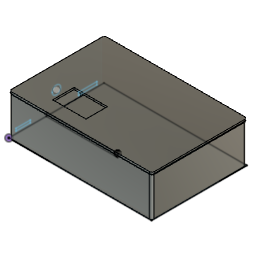
Ground Unit Enclosure v1.2 2 (Autodesk Fusion 360 design; units mm, degrees)
Autodesk Fusion 360 part; units mm, degrees
sketch "Sketch2" plane through (0, 0, 0) normal (0, 0, 1) x (1, 0, 0) in component "Case"
  line L0 (0, 0) -> (120, 0)
  line L1 (120, 0) -> (120, 80)
  line L2 (120, 80) -> (0, 80)
  line L3 (0, 80) -> (0, 0)
  dimension "d14" = 120
  dimension "d15" = 80
  constraint horizontal L0
  constraint vertical L1
  constraint horizontal L2
  constraint vertical L3
  constraint coincident L0.start L3.end
  measures "d14" distance of L0.start L0.end
  measures "d15" distance of L0.start L2.end
extrude "Extrude3" add sketch "Sketch2" along normal blind 33 makes body 1 in component "Case"
fillet "Fillet2" radius 2 1 edges at (120, 0, 16.5) on bodies 1 in component "Case"
fillet "Fillet3" radius 2 1 edges at (0, 0, 16.5) on bodies 1 in component "Case"
fillet "Fillet4" radius 2 2 edges at (120, 80, 16.5) (0, 80, 16.5) on bodies 1 in component "Case"
shell "Shell2" thickness 1.5 removed faces 1 at (40.6667, 26.6667, 33) on bodies 1 in component "Case"
sketch "Sketch Nub protrusion" plane through (0, 1.5, 0) normal (0, 1, 0) x (-1, 0, 0) in component "Case"
  line L0 (-2, 1.5) -> (-2, 33)
  line L1 (-2, 33) -> (-118, 33)
  line L2 (-118, 33) -> (-118, 1.5)
  line L3 (-118, 1.5) -> (-2, 1.5)
  line L4 (-90, 33) -> (-30, 33)
  line L5 (-30, 33) -> (-30, 30)
  line L6 (-30, 30) -> (-90, 30)
  line L7 (-90, 30) -> (-90, 33)
  line L8 (-60, 33) -> (-60, 30) construction
  dimension "d22" = 60
  dimension "d23" = 3
  constraint horizontal L4
  constraint vertical L5
  constraint horizontal L6
  constraint vertical L7
  constraint coincident L1 L4.start
  constraint midpoint L1 L8.start
  constraint midpoint L6 L8.end
  constraint vertical L8
  measures "d22" distance of L4.start L4.end
  measures "d23" distance of L4.start L6.end
extrude "Extrude4" add sketch "Sketch Nub protrusion" along normal blind 6 draft -45 contours L1 L4 L5 L6 L7 bodies 1 in component "Case"
ref_plane "WorkPlane1" through (60, 40, 16.5) normal (0, -1, 0) x (1, 0, 0) in component "Case"
mirror "Mirror1" about plane through (60, 40, 16.5) normal (0, -1, 0) of "Extrude4" in component "Case"
sketch "Sketch1" plane through (0, 0, 33) normal (0, 0, 1) x (-1, 0, 0) in component "Top Cover"
  arc A0 (-1.5, -2) -> (-2, -1.5) centre (-2, -2) ccw
  line L0 (-1.5, -2) -> (-1.5, -78)
  arc A1 (-2, -78.5) -> (-1.5, -78) centre (-2, -78) ccw
  line L1 (-2, -78.5) -> (-30, -78.5)
  line L2 (-30, -78.5) -> (-90, -78.5)
  line L3 (-90, -78.5) -> (-118, -78.5)
  arc A2 (-118.5, -78) -> (-118, -78.5) centre (-118, -78) ccw
  line L4 (-118.5, -78) -> (-118.5, -2)
  arc A3 (-118, -1.5) -> (-118.5, -2) centre (-118, -2) ccw
  line L5 (-118, -1.5) -> (-90, -1.5)
  line L6 (-90, -1.5) -> (-30, -1.5)
  line L7 (-30, -1.5) -> (-2, -1.5)
  arc A4 (-2, -80) -> (0, -78) centre (-2, -78) ccw
  line L8 (0, -78) -> (0, -2)
  arc A5 (0, -2) -> (-2, 0) centre (-2, -2) ccw
  line L9 (-2, 0) -> (-118, 0)
  arc A6 (-118, 0) -> (-120, -2) centre (-118, -2) ccw
  line L10 (-120, -2) -> (-120, -78)
  arc A7 (-120, -78) -> (-118, -80) centre (-118, -78) ccw
  line L11 (-118, -80) -> (-2, -80)
extrude "Extrude1" add sketch "Sketch1" along normal blind 2 separate body contours A0 L0 A1 L1 L2 L3 A2 L4 A3 L5 L6 L7 | A4 L8 A5 L9 A6 L10 A7 L11 makes body 2 in component "Top Cover"
sketch "Sketch2 (2)" plane through (0, 0, 33) normal (0, 0, -1) x (1, 0, 0) in component "Top Cover"
  line L0 (2, -80) -> (118, -80)
  arc A0 (118, -80) -> (120, -78) centre (118, -78) ccw
  line L1 (120, -78) -> (120, -2)
  arc A1 (120, -2) -> (118, 0) centre (118, -2) ccw
  line L2 (118, 0) -> (2, 0)
  arc A2 (2, 0) -> (0, -2) centre (2, -2) ccw
  line L3 (0, -2) -> (0, -78)
  arc A3 (0, -78) -> (2, -80) centre (2, -78) ccw
  arc A4 (1.7, -78) -> (2, -78.3) centre (2, -78) ccw
  line L4 (2, -78.3) -> (118, -78.3)
  arc A5 (118, -78.3) -> (118.3, -78) centre (118, -78) ccw
  line L5 (118.3, -78) -> (118.3, -2)
  arc A6 (118.3, -2) -> (118, -1.7) centre (118, -2) ccw
  line L6 (118, -1.7) -> (2, -1.7)
  arc A7 (2, -1.7) -> (1.7, -2) centre (2, -2) ccw
  line L7 (1.7, -2) -> (1.7, -78)
extrude "Extrude4'" add sketch "Sketch2 (2)" along normal blind 3 contours A4 L4 A5 L5 A6 L6 A7 L7 bodies 2 in component "Top Cover"
extrude "Extrude2" add sketch "Sketch2 (2)" along normal blind 3 contours A4 L4 A5 L5 A6 L6 A7 L7 bodies 2 in component "Top Cover"
extrude "Extrude3'" cut sketch "Sketch Nub protrusion" along normal blind 3 draft -45 from surface at 0.2 contours L1 L4 L5 L6 L7 bodies 2 in component "Top Cover"
mirror "Mirror1'" about plane through (60, 40, 16.5) normal (0, -1, 0) of "Extrude3'" in component "Top Cover"
shell "Shell1" thickness 1.5 removed faces 1 at (70, 52.7667, 30) on bodies 2 in component "Top Cover"
chamfer "Chamfer1" distance 0.6 angle 45 1 edges at (60, 78.3, 30) on bodies 2 in component "Top Cover"
chamfer "Chamfer2" distance 0.6 angle 45 1 edges at (60, 1.7, 30) on bodies 2 in component "Top Cover"
sketch "LCD Cutout" plane through (0, 0, 35) normal (0, 0, 1) x (-1, 0, 0) in component "Top Cover"
  line L0 (-118, -80) -> (-2, -80)
  arc A0 (-2, -80) -> (0, -78) centre (-2, -78) ccw
  line L1 (0, -78) -> (0, -2)
  arc A1 (0, -2) -> (-2, 0) centre (-2, -2) ccw
  line L2 (-2, 0) -> (-118, 0)
  arc A2 (-118, 0) -> (-120, -2) centre (-118, -2) ccw
  line L3 (-120, -2) -> (-120, -78)
  arc A3 (-120, -78) -> (-118, -80) centre (-118, -78) ccw
  line L4 (-24.9624, -29.5408) -> (-52.9624, -29.5408)
  line L5 (-52.9624, -29.5408) -> (-52.9624, -11.5408)
  line L6 (-52.9624, -11.5408) -> (-24.9624, -11.5408)
  line L7 (-24.9624, -11.5408) -> (-24.9624, -29.5408)
  dimension "d48" = 28
  dimension "d49" = 18
  constraint horizontal L4
  constraint vertical L5
  constraint horizontal L6
  constraint vertical L7
  measures "d48" distance of L4.start L4.end
  measures "d49" distance of L4.start L6.end
extrude "Extrude5" cut sketch "LCD Cutout" against normal blind 6 contours L4 L5 L6 L7 bodies 2 in component "Top Cover"
sketch "Ant Holes" plane through (0, 0, 0) normal (-1, 0, 0) x (0, -1, 0) in component "Case"
  line L0 (-78, 33) -> (-78, 0)
  line L1 (-78, 0) -> (-2, 0)
  line L2 (-2, 0) -> (-2, 33)
  line L3 (-2, 33) -> (-78, 33)
  circle A0 centre (-40, 15) radius 3.5
  line L4 (-18, 4) -> (-6, 4)
  line L5 (-6, 4) -> (-6, 2)
  line L6 (-6, 2) -> (-18, 2)
  line L7 (-18, 2) -> (-18, 4)
  line L8 (-74, 4) -> (-58.6271, 4)
  line L9 (-58.6271, 4) -> (-58.6271, 1.6206)
  line L10 (-58.6271, 1.6206) -> (-74, 1.6206)
  line L11 (-74, 1.6206) -> (-74, 4)
  dimension "d61" = 7
  constraint horizontal L4
  constraint vertical L5
  constraint horizontal L6
  constraint vertical L7
  constraint horizontal L8
  constraint vertical L9
  constraint horizontal L10
  constraint vertical L11
  measures "d61" diameter of A0
extrude "Extrude9" cut sketch "Ant Holes" against normal blind 7 contours L4 L5 L6 L7 bodies 1 in component "Case"
extrude "Extrude8" cut sketch "Ant Holes" against normal blind 7 contours A0 bodies 1 in component "Case"
extrude "Extrude10" cut sketch "Ant Holes" against normal blind 7 contours L8 L9 L10 L11 bodies 1 in component "Case"
extrude "Extrude11" add sketch "Ant Holes" against normal blind 7 contours L4 L5 L6 L7 bodies 1 in component "Case"
extrude "Extrude12" cut sketch "Ant Holes" against normal blind 7 contours L4 L5 L6 L7 bodies 1 in component "Case"
sketch "Sketch9" plane through (0, 0, 0) normal (0, 0, 1) x (1, 0, 0) in component "Case"
  circle A0 centre (55.0403, 35.9684) radius 2
  circle A1 centre (103.0403, 35.9069) radius 2
  dimension "d72" = 4
  dimension "d73" = 48
  dimension "d74" = 4
  measures "d72" diameter of A0
  measures "d73" distance of A0.centre A1.centre
  measures "d74" diameter of A1
extrude "Extrude13" cut sketch "Sketch9" along normal blind 7 bodies 1 in component "Case"
extrude "Extrude7" [suppressed] in component "Case"
extrude "Extrude6" [suppressed] in component "Case"
extrude "Extrude5'" [suppressed] in component "Case"
sketch "Sketch1 (2)" plane through (0, 0, 0) normal (0, 0, 1) x (1, 0, 0) in component "Case"
  line L0 (0, 0) -> (35, 0)
  line L1 (35, 0) -> (35, -50)
  line L2 (35, -50) -> (0, -50)
  line L3 (0, -50) -> (0, 0)
  dimension "d6" = 80
  dimension "d7" = 120
  constraint horizontal L0
  constraint vertical L1
  constraint horizontal L2
  constraint vertical L3
  constraint coincident L0.start L3.end
extrude "Extrude1'" [suppressed] in component "Case"
extrude "Extrude2'" [suppressed] in component "Case"
fillet "Fillet1" [suppressed] in component "Case"
shell "Shell1'" [suppressed] in component "Case"
component "Enclosure" placed x (1, 0, 0) y (0, 1, 0) z (0, 0, 1) at (0, 0, 0)
component "Case" placed x (1, 0, 0) y (0, 1, 0) z (0, 0, 1) at (0, 0, 0) in component "Enclosure"
component "Top Cover" placed x (1, 0, 0) y (0, 1, 0) z (0, 0, 1) at (0, 0, 0) in component "Enclosure"
equation "width = 80 mm"
equation "length = 120 mm"
equation "height = 33 mm"
equation "shell = 1.5 mm"
equation "gap = 0.2 mm"
equation "d6 = width"
equation "d7 = length"
equation "d8 = height"
equation "d10 = height"
equation "d13 = shell"
equation "d14 = length"
equation "d15 = width"
equation "d16 = height"
equation "d21 = shell"
equation "d22 = length / 2"
equation "d23 = shell * 2"
equation "d30 = -shell - gap"
equation "d31 = shell * 2"
equation "d34 = shell * 2"
equation "d36 = shell * 2"
equation "d40 = shell"
